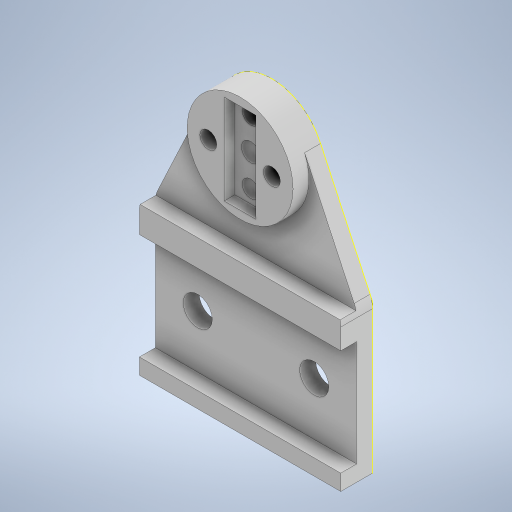
# Autodesk Inventor part: robot-arm-frame-base
Saved by Autodesk Inventor 2024.3 (Build 283343000, 343)
## iProperties
Created: 2024-11-17
Part Number: robot-arm-frame-base
Material: 一般
Document SubType Name: Modeling
Designer: azara
Density: 1 g/cm^3
Appearance: 既定
Author: azara
Autodesk Inventor part; units mm, degrees
ref_plane "YZ Plane" through (0, 0, 0) normal (1, 0, 0) x (0, 1, 0)
ref_plane "XZ Plane" through (0, 0, 0) normal (0, 1, 0) x (-1, 0, 0)
ref_plane "XY Plane" through (0, 0, 0) normal (0, 0, 1) x (1, 0, 0)
sketch "スケッチ1" plane through (0, 0, 0) normal (0, 0, 1) x (1, 0, 0)
  line L0 (0, 0) -> (38, 0)
  line L1 (38, 0) -> (38, 28)
  line L2 (0, 28) -> (0, 0)
  circle A0 centre (19, 45) radius 10
  line L3 (19, 45) -> (19, 0)
  line L4 (9, 45) -> (29, 45)
  line L5 (10.069714, 49.5) -> (27.930286, 49.5)
  line L6 (10.069714, 49.5) -> (0, 28)
  line L7 (27.930286, 49.5) -> (38, 28)
  point P0 (28.174131, 48.979363)
  point P1 (9.825869, 48.979363)
  dimension "d0" = 38
  dimension "d1" = 28
  dimension "d3" = 20
  dimension "d56" = 45
  dimension "d71" = 28
  dimension "d73" = 4.5
  constraints: 16 end point, 4 point on circle, 2 horizontal, 2 midpoint, 2 perpendicular, 1 centre point, 1 parallel
  measures "d0" distance of L0.start L0.end
  measures "d1" distance of L0.end L1.end
  measures "d3" diameter of A0
  measures "d56" distance of L3.start L3.end
  measures "d71" distance of L2.start L0.start
  measures "d73" distance from line of L5 L3.start
sketch "スケッチ1 outline for 押し出し1" plane through (0, 0, 0) normal (0, 0, 1) x (1, 0, 0)
  line L0 (9.825869, 48.979363) -> (0, 28)
  line L1 (0, 28) -> (0, 0)
  line L2 (0, 0) -> (38, 0)
  line L3 (38, 0) -> (38, 28)
  line L4 (38, 28) -> (28.174131, 48.979363)
  arc A0 (28.174131, 48.979363) -> (9.825869, 48.979363) centre (19, 45) ccw
extrude "押し出し1" add sketch "スケッチ1 outline for 押し出し1" along normal blind 3
sketch "スケッチ7" plane through (0, 0, 3) normal (0, 0, 1) x (1, 0, 0)
  line L0 (0, 0) -> (38, 0)
  line L1 (38, 0) -> (38, 28)
  line L2 (0, 0) -> (38, 0)
  line L3 (38, 0) -> (38, 3)
  line L4 (38, 3) -> (0, 3)
  line L5 (0, 3) -> (0, 0)
  arc A0 (28.174131, 48.979363) -> (9.825869, 48.979363) centre (19, 45) ccw
  circle A1 centre (19, 45) radius 10
  line L6 (0, 28) -> (0, 0)
  line L7 (0, 28) -> (38, 28)
  line L8 (38, 28) -> (38, 23)
  line L9 (38, 23) -> (0, 23)
  line L10 (0, 23) -> (0, 28)
  point P0 (27.930286, 47.5)
  point P1 (10.069714, 47.5)
  point P2 (0, 23)
  point P3 (29, 43)
  point P4 (9, 43)
  point P5 (10.069714, 47.5)
  point P6 (27.930286, 47.5)
  point P7 (9.486338, 51.080624)
  point P8 (28.513662, 51.080624)
  dimension "d58" = 3
  dimension "d68" = 20
  dimension "d69" = 20
  dimension "d70" = 5
  constraints: 16 end point, 4 parallel, 3 point on line, 2 horizontal, 2 perpendicular, 1 centre point, 1 coincident
  measures "d58" distance between parallel lines of L0 L4
  measures "d68" diameter of A1
  measures "d69" distance between parallel lines of L4 L9
  measures "d70" distance between parallel lines of L9 L7
extrude "押し出し4" add sketch "スケッチ7" along normal blind 3 contours L5 L4 L1 L0 | L6 L7 L1 L9 | A1 A0
sketch "スケッチ10" plane through (19, 45, 6) normal (0, 0, 1) x (1, 0, 0)
  line L0 (-3, 8.5) -> (3, 8.5)
  line L1 (3, 8.5) -> (3, -8.5)
  line L2 (3, -8.5) -> (-3, -8.5)
  line L3 (-3, -8.5) -> (-3, 8.5)
  circle A0 centre (0, 0) radius 10 projected
  point P0 (-19, -45)
  dimension "d74" = 8.5
  dimension "d75" = 17
  dimension "d76" = 6
  dimension "d77" = 3
  constraints: 8 end point, 2 parallel, 1 horizontal, 1 perpendicular
  measures "d74" distance from line of A0.centre L0
  measures "d75" distance of L2.end L0.start
  measures "d76" distance of L0.start L0.end
  measures "d77" distance from line of L1 A0.centre
extrude "押し出し7" cut sketch "スケッチ10" against normal blind 2 contours L0 L1 L2 L3
sketch "スケッチ11" plane through (0, 0, 0) normal (0, 0, -1) x (-1, 0, 0)
  arc A0 (-9.825869, 48.979363) -> (-28.174131, 48.979363) centre (-19, 45) ccw
  point P0 (0, 0)
  point P1 (-27.930286, 47.5)
  point P2 (-10.069714, 47.5)
  point P3 (-19, 51)
  point P4 (-25, 45)
  point P5 (-19, 39)
  point P6 (-13, 45)
  dimension "d80" = 6
  dimension "d83" = 360
  constraints: 5 other
  measures "d80" distance of A0.centre point (-19, 51)
hole "穴4" at (19, 51, 0) at (25, 45, 0) at (19, 39, 0) at (13, 45, 0) direction (0, 0, 1) diameter 3.2 end through all
sketch "スケッチ12" plane through (0, 0, 0) normal (0, 0, -1) x (-1, 0, 0)
  circle A0 centre (-19, 45) radius 10 projected
  point P0 (0, 0)
  constraints: 1 coincident
hole "穴5" at (19, 45, 0) direction (0, 0, 1) diameter 3.5 end through all
sketch "スケッチ13" plane through (0, 0, 0) normal (0, 0, -1) x (-1, 0, 0)
  circle A0 centre (-19, 45) radius 1.75
  circle A1 centre (-13, 45) radius 1.6
  circle A2 centre (-19, 39) radius 1.6
  circle A3 centre (-25, 45) radius 1.6
  circle A4 centre (-19, 51) radius 1.6
  arc A5 (-9.825869, 48.979363) -> (-28.174131, 48.979363) centre (-19, 45) ccw
  line L0 (-38, 28) -> (-28.174131, 48.979363)
  line L1 (-38, 0) -> (-38, 28)
  line L2 (0, 0) -> (-38, 0)
  line L3 (0, 28) -> (0, 0)
  line L4 (-9.825869, 48.979363) -> (0, 28)
fillet "フィレット1" radius 5 2 edges at (0, 28, 1.5) (38, 28, 1.5)
sketch "スケッチ14" plane through (0, 0, 3) normal (0, 0, 1) x (1, 0, 0)
  line L0 (0, 0) -> (38, 0) projected
  line L1 (0, 23) -> (0, 3) projected
  line L2 (38, 3) -> (38, 23) projected
  point P0 (8, 13)
  point P1 (30, 13)
  dimension "d100" = 13
  dimension "d101" = 13
  dimension "d102" = 8
  dimension "d103" = 8
  measures "d100" distance from line of L0 point (8, 13)
  measures "d101" distance from line of L0 point (30, 13)
  measures "d102" distance from line of L1 point (8, 13)
  measures "d103" distance from line of point (30, 13) L2
hole "穴6" at (8, 13, 3) at (30, 13, 3) direction (0, 0, -1) diameter 5.5 end through all
